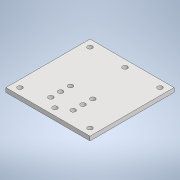
# Autodesk Inventor part: Lift.00.00.00.01
Saved by Autodesk Inventor 2021 (Build 250183000, 183)
## iProperties
Created: 2020-09-20
Part Number: Lift.00.00.00.01
Material: Типовые
Document SubType Name: ЛистМат
Designer: Kostya
Density: 1 g/cm^3
Sheet Metal Rule: По умолчанию_мм
Appearance: По умолчанию
Author: Kostya
Autodesk Inventor part; units mm, degrees
ref_plane "YZ Plane" through (0, 0, 0) normal (1, 0, 0) x (0, 1, 0)
ref_plane "XZ Plane" through (0, 0, 0) normal (0, 1, 0) x (-1, 0, 0)
ref_plane "XY Plane" through (0, 0, 0) normal (0, 0, 1) x (1, 0, 0)
sketch "Эскиз1" plane through (0, 0, 0) normal (0, 1, 0) x (-1, 0, 0)
  line L0 (-150, 150) -> (150, 150)
  line L1 (150, 150) -> (150, -150)
  line L2 (150, -150) -> (-150, -150)
  line L3 (-150, -150) -> (-150, 150)
  line L4 (-150, 150) -> (150, -150) construction
  line L5 (150, 150) -> (-150, -150) construction
  circle A0 centre (125, -125) radius 8.5
  circle A1 centre (0, -125) radius 8.5
  circle A2 centre (-125, -125) radius 8.5
  circle A3 centre (125, 125) radius 8.5
  circle A4 centre (0, 125) radius 8.5
  circle A5 centre (40, 100) radius 8.5
  circle A6 centre (40, 65) radius 8.5
  circle A7 centre (40, 30) radius 8.5
  circle A8 centre (-40, 30) radius 8.5
  circle A9 centre (-40, 65) radius 8.5
  circle A10 centre (-40, 100) radius 8.5
  circle A11 centre (-125, -125) radius 8.5
  circle A12 centre (-125, 125) radius 8.5
  point P0 (0, 0)
  point P1 (0, 0)
  point P2 (0, 0)
  dimension "d0" = 300
  dimension "d1" = 300
  dimension "d2" = 17
  dimension "d3" = 50
  dimension "d4" = 85
  dimension "d5" = 120
  dimension "d6" = 80
  dimension "d7" = 40
  dimension "d8" = 25
  dimension "d9" = 25
  dimension "d10" = 25
  dimension "d11" = 25
  measures "d0" distance of L1.end L2.end
  measures "d1" distance of L0.end L1.end
  measures "d2" diameter of A2
  measures "d3" distance from line of L0 A10.centre
  measures "d4" distance from line of L0 A9.centre
  measures "d5" distance from line of L0 A8.centre
  measures "d6" distance of A7.centre A8.centre
  measures "d7" horizontal distance of point (0, 0) A8.centre
  measures "d8" distance from line of L2 A0.centre
  measures "d9" distance from line of L1 A0.centre
  measures "d10" distance from line of L3 A2.centre
  measures "d11" distance from line of L0 A12.centre
extrude "Пластина1" add sketch "Эскиз1" along normal blind 15
equation "\"d12\" = Толщина"
equation "\"Радиус_гибки\" = Толщина"
equation "\"Ширина_просечки\" = Толщина"
equation "\"Глубина_просечки\" = 0.5 * Толщина"
equation "\"Радиус_перехода\" = Радиус_гибки"
equation "\"Радиус_Якоби\" = Радиус_гибки"
equation "\"Размер_зазора\" = Толщина"
equation "\"Толщина\" = 15"
